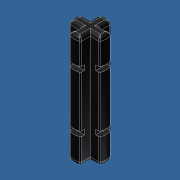
# Autodesk Inventor part: 32062
Saved by Autodesk Inventor 2011 SP2 (Build 150553200, 553)
## iProperties
Company: Allseas Engineering BV
Created: 2011-11-29
Part Number: 32062
Cost Center: 0 kg
Material: Steel
Document SubType Name: Modeling
Designer: PMe
Authority: 0 mm^3
Stock Number: =<Filenr>_<Document number>
Mass: 1.4258 g
Surface Area: 2.99966 cm^2
Volume: 0.18163 cm^3
Density: 7.85 g/cm^3
Act. Code: DW000
SaveDate: 2011-07-28
SaveTime: 18:32
FileName: Standard
TotalMass: 0 kg
TotalVolume: 0 mm^3
Subject: =<Title><TITLE 1_2> <TITLE 2_2>
Author: PMe
Autodesk Inventor part; units mm, degrees
ref_plane "YZ Plane" through (0, 0, 0) normal (1, 0, 0) x (0, 1, 0)
ref_plane "XZ Plane" through (0, 0, 0) normal (0, 1, 0) x (-1, 0, 0)
ref_plane "XY Plane" through (0, 0, 0) normal (0, 0, 1) x (1, 0, 0)
sketch "Sketch1" plane through (0, 0, 0) normal (0, 0, 1) x (1, 0, 0)
  circle A0 centre (0, 0) radius 2.3
  line L0 (-2.1564, 0.8) -> (-0.8, 0.8)
  line L1 (-0.8, 0.8) -> (-0.8, 2.1564)
  line L2 (0.8, 2.1564) -> (0.8, 0.8)
  line L3 (0.8, 0.8) -> (2.1564, 0.8)
  line L4 (2.1564, -0.8) -> (0.8, -0.8)
  line L5 (0.8, -0.8) -> (0.8, -2.1564)
  line L6 (-0.8, -2.1564) -> (-0.8, -0.8)
  line L7 (-0.8, -0.8) -> (-2.1564, -0.8)
  dimension "d0" = 4.6
  dimension "d1" = 1.6
  constraints: 16 end point, 4 perpendicular, 3 equal length, 3 parallel, 2 horizontal alignment, 2 vertical alignment, 1 coincident, 1 horizontal, 10 other
  measures "d1" distance between parallel lines of L2 L1
extrude "Extrusion1" add sketch "Sketch1" along normal mid plane 16 contours A0 L4 L5 L6 L7 L0 L1 L2 L3
fillet "Fillet1" radius 0.5 24 edges at (0, 2.3, 8) (0.8, 1.4782, 8) (1.4782, 0.8, 8) (2.3, 0, 8) (1.4782, -0.8, 8) (0.8, -1.4782, 8) (0, -2.3, 8) (-0.8, -1.4782, 8) (-1.4782, -0.8, 8) (-2.3, 0, 8) (-1.4782, 0.8, 8) (-0.8, 1.4782, 8) (0, 2.3, -8) (-2.3, 0, -8) (0, -2.3, -8) (2.3, 0, -8) (1.4782, 0.8, -8) (0.8, 1.4782, -8) (-0.8, 1.4782, -8) (-1.4782, 0.8, -8) (-1.4782, -0.8, -8) (-0.8, -1.4782, -8) (0.8, -1.4782, -8) (1.4782, -0.8, -8)
fillet "Fillet2" radius 0.2 24 edges at (0.8, 2.1564, 0) (0.6467, 2.047, 7.8603) (0.6467, 2.047, -7.8603) (-0.8, 2.1564, 0) (-0.6467, 2.047, 7.8603) (-0.6467, 2.047, -7.8603) (-2.1564, 0.8, 0) (-2.047, 0.6467, -7.8603) (-2.047, 0.6467, 7.8603) (-2.1564, -0.8, 0) (-2.047, -0.6467, 7.8603) (-2.047, -0.6467, -7.8603) (-0.8, -2.1564, 0) (-0.6467, -2.047, 7.8603) (-0.6467, -2.047, -7.8603) (0.8, -2.1564, 0) (0.6467, -2.047, 7.8603) (0.6467, -2.047, -7.8603) (2.1564, -0.8, 0) (2.047, -0.6467, 7.8603) (2.047, -0.6467, -7.8603) (2.1564, 0.8, 0) (2.047, 0.6467, 7.8603) (2.047, 0.6467, -7.8603)
sketch "Sketch2" plane through (-0.8, 0.8, -7.5) normal (-1, 0, 0) x (0, 0, 1)
  line L0 (0, 1.5) -> (0, 1.4041) projected
  line L1 (15, 1.4041) -> (15, 1.5) projected
  line L2 (0, 1.5) -> (15, 1.5)
  line L3 (3.15, 1.5) -> (3.15, 0.8)
  line L4 (3.15, 0.8) -> (3.85, 0.8)
  line L5 (3.85, 0.8) -> (3.85, 1.5)
  line L6 (-0.5, 0.9748) -> (-0.5, -0.5) projected
  line L7 (11.15, 1.5) -> (11.85, 1.5)
  line L8 (11.85, 1.5) -> (11.85, 0.8)
  line L9 (11.85, 0.8) -> (11.15, 0.8)
  line L10 (11.15, 0.8) -> (11.15, 1.5)
  line L11 (15.5, -0.5) -> (15.5, 0.9748) projected
  point P0 (7.5, -0.8)
  dimension "d6" = 0.7
  dimension "d7" = 0.7
  dimension "d8" = 3.65
  dimension "d9" = 3.65
  constraints: 16 end point, 5 perpendicular, 3 point on line, 2 equal length, 2 parallel, 1 horizontal
  measures "d6" distance of L3.start L3.end
  measures "d7" distance of L3.end L4.end
  measures "d8" distance between parallel lines of L6 L3
  measures "d9" distance between parallel lines of L11 L8
extrude "Extrusion2" cut sketch "Sketch2" against normal up to surface (1.6 mm away)
pattern_circular "Circular Pattern1" count 4 over 360 about axis through (0, 0, -10) along (0, 0, 1) of "Extrusion2"
equation "\"d9\" = d8"
body "Solid1"
